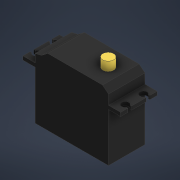
# Autodesk Inventor part: Servo
Saved by Autodesk Inventor 2021 (Build 250183000, 183)
## iProperties
Created: 2021-01-09
Part Number: Servo
Material: Generisch
Document SubType Name: Modeling
Designer: laure
Density: 1 g/cm^3
Appearance: Vorgabe
Author: laure
Autodesk Inventor part; units mm, degrees
ref_plane "YZ Plane" through (0, 0, 0) normal (1, 0, 0) x (0, 1, 0)
ref_plane "XZ Plane" through (0, 0, 0) normal (0, 1, 0) x (-1, 0, 0)
ref_plane "XY Plane" through (0, 0, 0) normal (0, 0, 1) x (1, 0, 0)
sketch "Skizze1" plane through (0, 0, 0) normal (0, 0, 1) x (1, 0, 0)
  line L0 (-20.15, 13.3) -> (20.15, 13.3)
  line L1 (20.15, 13.3) -> (20.15, -13.3)
  line L2 (20.15, -13.3) -> (-20.15, -13.3)
  line L3 (-20.15, -13.3) -> (-20.15, 13.3)
  line L4 (0, 30.62) -> (0, -20.62) projected
  line L5 (-37.52, 0) -> (37.52, 0) projected
  line L6 (-20.15, 13.3) -> (-20.15, 19.8141)
  line L7 (-13.1284, 23.3) -> (16.9083, 23.3)
  line L8 (20.15, 20.6722) -> (20.15, 13.3)
  line L9 (16.9083, 23.3) -> (20.15, 20.6722)
  line L10 (-20.15, 19.8141) -> (-16.5313, 20.6722)
  line L11 (-16.5313, 20.6722) -> (-13.1284, 23.3)
  line L12 (20.15, 13.3) -> (26.8, 13.3)
  line L13 (26.8, 13.3) -> (26.8, 15.3)
  line L14 (26.8, 15.3) -> (20.15, 15.3)
  line L15 (20.15, 15.3) -> (20.15, 13.3)
  line L16 (-20.15, 13.3) -> (-26.8, 13.3)
  line L17 (-26.8, 13.3) -> (-26.8, 15.3)
  line L18 (-26.8, 15.3) -> (-20.15, 15.3)
  line L19 (-20.15, 15.3) -> (-20.15, 13.3)
  line L20 (6, 23.3) -> (11, 23.3)
  point P0 (0, 0)
  dimension "d0" = 40.3
  dimension "d1" = 26.6
  dimension "d3" = 10
  dimension "d4" = 3.6187
  dimension "d5" = 3.4029
  dimension "d6" = 3.2417
  dimension "d7" = 103.34
  dimension "d8" = 142.325
  dimension "d9" = 140.972
  dimension "d10" = 6.65
  dimension "d11" = 2
  dimension "d12" = 6.65
  dimension "d13" = 2
  constraints: 38 end point, 6 parallel, 5 perpendicular, 4 horizontal, 1 point on line, 2 other
  measures "d0" distance of L1.end L2.end
  measures "d1" distance between parallel lines of L2 L0
  measures "d3" distance between parallel lines of L7 L0
  measures "d4" horizontal distance of L10.end L6.end
  measures "d5" horizontal distance of L7.start L10.end
  measures "d6" horizontal distance of L8.start L7.end
  measures "d7" angle of L6 L10
  measures "d8" angle of L7 L11
  measures "d9" angle of L7 L9
  measures "d10" distance of L14.end L13.end
  measures "d11" distance of L13.end L12.end
  measures "d12" distance of L17.end L18.end
  measures "d13" distance of L16.end L17.end
extrude "Extrusion1" add sketch "Skizze1" along normal mid plane 20
sketch "Skizze2" plane through (-26.8, 15.3, 10) normal (0, 1, 0) x (1, 0, 0)
  line L0 (64.32, 10) -> (-10.72, 10) projected
  line L1 (26.8, 24) -> (26.8, -4) projected
  arc A0 (0.7679, 14) -> (0.7679, 16) centre (2.5, 15) ccw
  line L2 (0, 20) -> (0, 0) projected
  line L3 (0.7679, 16) -> (0, 16)
  line L4 (0, 20) -> (0, 0) projected
  line L5 (0.7679, 14) -> (0, 14)
  line L6 (0, 16) -> (0, 14)
  line L7 (2.5, 15) -> (0.8619, 15)
  arc A1 (0.7679, 4) -> (0.7679, 6) centre (2.5, 5) ccw
  line L8 (0.7679, 4) -> (0, 4)
  line L9 (0.7679, 6) -> (0, 6)
  line L10 (0, 4) -> (0, 6)
  line L11 (2.5, 5) -> (0.8619, 5)
  arc A2 (52.8321, 16) -> (52.8321, 14) centre (51.1, 15) ccw
  line L12 (52.8321, 16) -> (53.6, 16)
  line L13 (52.8321, 14) -> (53.6, 14)
  line L14 (53.6, 16) -> (53.6, 14)
  line L15 (51.1, 15) -> (52.7381, 15)
  arc A3 (52.8321, 6) -> (52.8321, 4) centre (51.1, 5) ccw
  line L16 (52.8321, 4) -> (53.6, 4)
  line L17 (52.8321, 6) -> (53.6, 6)
  line L18 (53.6, 4) -> (53.6, 6)
  line L19 (51.1, 5) -> (52.7381, 5)
  point P0 (26.8, 10)
  dimension "d19" = 4
  dimension "d21" = 5
  dimension "d23" = 2.5
  dimension "d25" = 2
  constraints: 32 end point, 18 symmetric about line, 8 point on circle, 4 centre point, 2 perpendicular, 2 point on line, 1 collinear, 1 horizontal, 4 other
  measures "d19" diameter of A0
  measures "d21" distance from line of L0 L7.start
  measures "d23" distance from line of L7.start L2
  measures "d25" distance between parallel lines of L3 L5
extrude "Extrusion2" cut sketch "Skizze2" against normal up to surface (2 mm away)
sketch "Skizze3" plane through (-13.1284, 23.3, 10) normal (0, 1, 0) x (1, 0, 0)
  line L0 (13.1284, 24) -> (13.1284, -4) projected
  line L1 (-24.3916, 10) -> (50.6484, 10) projected
  circle A0 centre (23.1284, 10) radius 3
  point P0 (13.1284, 10)
  dimension "d28" = 6
  dimension "d29" = 10
  constraints: 1 centre point, 1 point on line
  measures "d28" diameter of A0
  measures "d29" distance from line of A0.centre L0
extrude "Extrusion3" add sketch "Skizze3" along normal blind 5
